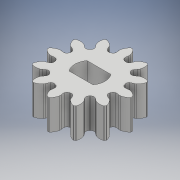
# Autodesk Inventor part: RescueKit-Gear-8
Saved by Autodesk Inventor 2018.3 (Build 223284000, 284)
## iProperties
Created: 2019-03-13
Part Number: RescueKit-Gear-8
Material: 一般
Document SubType Name: Modeling
Designer: shun2
Density: 1 g/cm^3
Appearance: 既定
Author: shun2
Autodesk Inventor part; units mm, degrees
ref_plane "YZ Plane" through (0, 0, 0) normal (1, 0, 0) x (0, 1, 0)
ref_plane "XZ Plane" through (0, 0, 0) normal (0, 1, 0) x (-1, 0, 0)
ref_plane "XY Plane" through (0, 0, 0) normal (0, 0, 1) x (1, 0, 0)
sketch "スケッチ1" plane through (0, 0, 0) normal (0, 0, 1) x (1, 0, 0)
  arc A0 (-0.202, 6.9715) -> (-0.7832, 5.9487) centre (1.1694, 5.5158) ccw
  arc A1 (-0.1354, 6.9987) -> (-0.202, 6.9715) centre (-0.1335, 6.8987) ccw
  arc A2 (0.1354, 6.9987) -> (-0.1354, 6.9987) centre (0, 0) ccw
  arc A3 (0.202, 6.9715) -> (0.1354, 6.9987) centre (0.1335, 6.8987) ccw
  arc A4 (0.7832, 5.9487) -> (0.202, 6.9715) centre (-1.1694, 5.5158) ccw
  arc A5 (0.7831, 5.6009) -> (0.7832, 5.9487) centre (0, 5.775) ccw
  arc A6 (0.7831, 5.6009) -> (0.7441, 5.0639) centre (2.5852, 5.2003) ccw
  arc A7 (0.7441, 5.0639) -> (1.1244, 4.615) centre (1.2427, 5.1008) ccw
  arc A8 (1.3338, 4.5589) -> (1.1244, 4.615) centre (0, 0) ccw
  arc A9 (1.3338, 4.5589) -> (1.8875, 4.7575) centre (1.4742, 5.0388) ccw
  arc A10 (1.8875, 4.7575) -> (2.1223, 5.2421) centre (0.3613, 5.7962) ccw
  arc A11 (2.2961, 5.5433) -> (2.1223, 5.2421) centre (2.8875, 5.0013) ccw
  arc A12 (3.3108, 6.1385) -> (2.2961, 5.5433) centre (3.7707, 4.1921) ccw
  arc A13 (3.3821, 6.1287) -> (3.3108, 6.1385) centre (3.3338, 6.0412) ccw
  arc A14 (3.6166, 5.9933) -> (3.3821, 6.1287) centre (0, 0) ccw
  arc A15 (3.6607, 5.9365) -> (3.6166, 5.9933) centre (3.5649, 5.9077) ccw
  arc A16 (3.6526, 4.7601) -> (3.6607, 5.9365) centre (1.7451, 5.3615) ccw
  arc A17 (3.4786, 4.459) -> (3.6526, 4.7601) centre (2.8875, 5.0013) ccw
  arc A18 (3.4786, 4.459) -> (3.1763, 4.0134) centre (4.839, 3.211) ccw
  arc A19 (3.1763, 4.0134) -> (3.2812, 3.4345) centre (3.6266, 3.7961) ccw
  arc A20 (3.4345, 3.2812) -> (3.2812, 3.4345) centre (0, 0) ccw
  arc A21 (3.4345, 3.2812) -> (4.0134, 3.1763) centre (3.7961, 3.6266) ccw
  arc A22 (4.0134, 3.1763) -> (4.459, 3.4786) centre (3.211, 4.839) ccw
  arc A23 (4.7601, 3.6526) -> (4.459, 3.4786) centre (5.0013, 2.8875) ccw
  arc A24 (5.9365, 3.6607) -> (4.7601, 3.6526) centre (5.3615, 1.7451) ccw
  arc A25 (5.9933, 3.6166) -> (5.9365, 3.6607) centre (5.9077, 3.5649) ccw
  arc A26 (6.1287, 3.3821) -> (5.9933, 3.6166) centre (0, 0) ccw
  arc A27 (6.1385, 3.3108) -> (6.1287, 3.3821) centre (6.0412, 3.3338) ccw
  arc A28 (5.5433, 2.2961) -> (6.1385, 3.3108) centre (4.1921, 3.7707) ccw
  arc A29 (5.2421, 2.1223) -> (5.5433, 2.2961) centre (5.0013, 2.8875) ccw
  arc A30 (5.2421, 2.1223) -> (4.7575, 1.8875) centre (5.7962, 0.3613) ccw
  arc A31 (4.7575, 1.8875) -> (4.5589, 1.3338) centre (5.0388, 1.4742) ccw
  arc A32 (4.615, 1.1244) -> (4.5589, 1.3338) centre (0, 0) ccw
  arc A33 (4.615, 1.1244) -> (5.0639, 0.7441) centre (5.1008, 1.2427) ccw
  arc A34 (5.0639, 0.7441) -> (5.6009, 0.7831) centre (5.2003, 2.5852) ccw
  arc A35 (5.9487, 0.7832) -> (5.6009, 0.7831) centre (5.775, 0) ccw
  arc A36 (6.9715, 0.202) -> (5.9487, 0.7832) centre (5.5158, -1.1694) ccw
  arc A37 (6.9987, 0.1354) -> (6.9715, 0.202) centre (6.8987, 0.1335) ccw
  arc A38 (6.9987, -0.1354) -> (6.9987, 0.1354) centre (0, 0) ccw
  arc A39 (6.9715, -0.202) -> (6.9987, -0.1354) centre (6.8987, -0.1335) ccw
  arc A40 (5.9487, -0.7832) -> (6.9715, -0.202) centre (5.5158, 1.1694) ccw
  arc A41 (5.6009, -0.7831) -> (5.9487, -0.7832) centre (5.775, 0) ccw
  arc A42 (5.6009, -0.7831) -> (5.0639, -0.7441) centre (5.2003, -2.5852) ccw
  arc A43 (5.0639, -0.7441) -> (4.615, -1.1244) centre (5.1008, -1.2427) ccw
  arc A44 (4.5589, -1.3338) -> (4.615, -1.1244) centre (0, 0) ccw
  arc A45 (4.5589, -1.3338) -> (4.7575, -1.8875) centre (5.0388, -1.4742) ccw
  arc A46 (4.7575, -1.8875) -> (5.2421, -2.1223) centre (5.7962, -0.3613) ccw
  arc A47 (5.5433, -2.2961) -> (5.2421, -2.1223) centre (5.0013, -2.8875) ccw
  arc A48 (6.1385, -3.3108) -> (5.5433, -2.2961) centre (4.1921, -3.7707) ccw
  arc A49 (6.1287, -3.3821) -> (6.1385, -3.3108) centre (6.0412, -3.3338) ccw
  arc A50 (5.9933, -3.6166) -> (6.1287, -3.3821) centre (0, 0) ccw
  arc A51 (5.9365, -3.6607) -> (5.9933, -3.6166) centre (5.9077, -3.5649) ccw
  arc A52 (4.7601, -3.6526) -> (5.9365, -3.6607) centre (5.3615, -1.7451) ccw
  arc A53 (4.459, -3.4786) -> (4.7601, -3.6526) centre (5.0013, -2.8875) ccw
  arc A54 (4.459, -3.4786) -> (4.0134, -3.1763) centre (3.211, -4.839) ccw
  arc A55 (4.0134, -3.1763) -> (3.4345, -3.2812) centre (3.7961, -3.6266) ccw
  arc A56 (3.2812, -3.4345) -> (3.4345, -3.2812) centre (0, 0) ccw
  arc A57 (3.2812, -3.4345) -> (3.1763, -4.0134) centre (3.6266, -3.7961) ccw
  arc A58 (3.1763, -4.0134) -> (3.4786, -4.459) centre (4.839, -3.211) ccw
  arc A59 (3.6526, -4.7601) -> (3.4786, -4.459) centre (2.8875, -5.0013) ccw
  arc A60 (3.6607, -5.9365) -> (3.6526, -4.7601) centre (1.7451, -5.3615) ccw
  arc A61 (3.6166, -5.9933) -> (3.6607, -5.9365) centre (3.5649, -5.9077) ccw
  arc A62 (3.3821, -6.1287) -> (3.6166, -5.9933) centre (0, 0) ccw
  arc A63 (3.3108, -6.1385) -> (3.3821, -6.1287) centre (3.3338, -6.0412) ccw
  arc A64 (2.2961, -5.5433) -> (3.3108, -6.1385) centre (3.7707, -4.1921) ccw
  arc A65 (2.1223, -5.2421) -> (2.2961, -5.5433) centre (2.8875, -5.0013) ccw
  arc A66 (2.1223, -5.2421) -> (1.8875, -4.7575) centre (0.3613, -5.7962) ccw
  arc A67 (1.8875, -4.7575) -> (1.3338, -4.5589) centre (1.4742, -5.0388) ccw
  arc A68 (1.1244, -4.615) -> (1.3338, -4.5589) centre (0, 0) ccw
  arc A69 (1.1244, -4.615) -> (0.7441, -5.0639) centre (1.2427, -5.1008) ccw
  arc A70 (0.7441, -5.0639) -> (0.7831, -5.6009) centre (2.5852, -5.2003) ccw
  arc A71 (0.7832, -5.9487) -> (0.7831, -5.6009) centre (0, -5.775) ccw
  arc A72 (0.202, -6.9715) -> (0.7832, -5.9487) centre (-1.1694, -5.5158) ccw
  arc A73 (0.1354, -6.9987) -> (0.202, -6.9715) centre (0.1335, -6.8987) ccw
  arc A74 (-0.1354, -6.9987) -> (0.1354, -6.9987) centre (0, 0) ccw
  arc A75 (-0.202, -6.9715) -> (-0.1354, -6.9987) centre (-0.1335, -6.8987) ccw
  arc A76 (-0.7832, -5.9487) -> (-0.202, -6.9715) centre (1.1694, -5.5158) ccw
  arc A77 (-0.7831, -5.6009) -> (-0.7832, -5.9487) centre (0, -5.775) ccw
  arc A78 (-0.7831, -5.6009) -> (-0.7441, -5.0639) centre (-2.5852, -5.2003) ccw
  arc A79 (-0.7441, -5.0639) -> (-1.1244, -4.615) centre (-1.2427, -5.1008) ccw
  arc A80 (-1.3338, -4.5589) -> (-1.1244, -4.615) centre (0, 0) ccw
  arc A81 (-1.3338, -4.5589) -> (-1.8875, -4.7575) centre (-1.4742, -5.0388) ccw
  arc A82 (-1.8875, -4.7575) -> (-2.1223, -5.2421) centre (-0.3613, -5.7962) ccw
  arc A83 (-2.2961, -5.5433) -> (-2.1223, -5.2421) centre (-2.8875, -5.0013) ccw
  arc A84 (-3.3108, -6.1385) -> (-2.2961, -5.5433) centre (-3.7707, -4.1921) ccw
  arc A85 (-3.3821, -6.1287) -> (-3.3108, -6.1385) centre (-3.3338, -6.0412) ccw
  arc A86 (-3.6166, -5.9933) -> (-3.3821, -6.1287) centre (0, 0) ccw
  arc A87 (-3.6607, -5.9365) -> (-3.6166, -5.9933) centre (-3.5649, -5.9077) ccw
  arc A88 (-3.6526, -4.7601) -> (-3.6607, -5.9365) centre (-1.7451, -5.3615) ccw
  arc A89 (-3.4786, -4.459) -> (-3.6526, -4.7601) centre (-2.8875, -5.0013) ccw
  arc A90 (-3.4786, -4.459) -> (-3.1763, -4.0134) centre (-4.839, -3.211) ccw
  arc A91 (-3.1763, -4.0134) -> (-3.2812, -3.4345) centre (-3.6266, -3.7961) ccw
  arc A92 (-3.4345, -3.2812) -> (-3.2812, -3.4345) centre (0, 0) ccw
  arc A93 (-3.4345, -3.2812) -> (-4.0134, -3.1763) centre (-3.7961, -3.6266) ccw
  arc A94 (-4.0134, -3.1763) -> (-4.459, -3.4786) centre (-3.211, -4.839) ccw
  arc A95 (-4.7601, -3.6526) -> (-4.459, -3.4786) centre (-5.0013, -2.8875) ccw
  arc A96 (-5.9365, -3.6607) -> (-4.7601, -3.6526) centre (-5.3615, -1.7451) ccw
  arc A97 (-5.9933, -3.6166) -> (-5.9365, -3.6607) centre (-5.9077, -3.5649) ccw
  arc A98 (-6.1287, -3.3821) -> (-5.9933, -3.6166) centre (0, 0) ccw
  arc A99 (-6.1385, -3.3108) -> (-6.1287, -3.3821) centre (-6.0412, -3.3338) ccw
  arc A100 (-5.5433, -2.2961) -> (-6.1385, -3.3108) centre (-4.1921, -3.7707) ccw
  arc A101 (-5.2421, -2.1223) -> (-5.5433, -2.2961) centre (-5.0013, -2.8875) ccw
  arc A102 (-5.2421, -2.1223) -> (-4.7575, -1.8875) centre (-5.7962, -0.3613) ccw
  arc A103 (-4.7575, -1.8875) -> (-4.5589, -1.3338) centre (-5.0388, -1.4742) ccw
  arc A104 (-4.615, -1.1244) -> (-4.5589, -1.3338) centre (0, 0) ccw
  arc A105 (-4.615, -1.1244) -> (-5.0639, -0.7441) centre (-5.1008, -1.2427) ccw
  arc A106 (-5.0639, -0.7441) -> (-5.6009, -0.7831) centre (-5.2003, -2.5852) ccw
  arc A107 (-5.9487, -0.7832) -> (-5.6009, -0.7831) centre (-5.775, 0) ccw
  arc A108 (-6.9715, -0.202) -> (-5.9487, -0.7832) centre (-5.5158, 1.1694) ccw
  arc A109 (-6.9987, -0.1354) -> (-6.9715, -0.202) centre (-6.8987, -0.1335) ccw
  arc A110 (-6.9987, 0.1354) -> (-6.9987, -0.1354) centre (0, 0) ccw
  arc A111 (-6.9715, 0.202) -> (-6.9987, 0.1354) centre (-6.8987, 0.1335) ccw
  arc A112 (-5.9487, 0.7832) -> (-6.9715, 0.202) centre (-5.5158, -1.1694) ccw
  arc A113 (-5.6009, 0.7831) -> (-5.9487, 0.7832) centre (-5.775, 0) ccw
  arc A114 (-5.6009, 0.7831) -> (-5.0639, 0.7441) centre (-5.2003, 2.5852) ccw
  arc A115 (-5.0639, 0.7441) -> (-4.615, 1.1244) centre (-5.1008, 1.2427) ccw
  arc A116 (-4.5589, 1.3338) -> (-4.615, 1.1244) centre (0, 0) ccw
  arc A117 (-4.5589, 1.3338) -> (-4.7575, 1.8875) centre (-5.0388, 1.4742) ccw
  arc A118 (-4.7575, 1.8875) -> (-5.2421, 2.1223) centre (-5.7962, 0.3613) ccw
  arc A119 (-5.5433, 2.2961) -> (-5.2421, 2.1223) centre (-5.0013, 2.8875) ccw
  arc A120 (-6.1385, 3.3108) -> (-5.5433, 2.2961) centre (-4.1921, 3.7707) ccw
  arc A121 (-6.1287, 3.3821) -> (-6.1385, 3.3108) centre (-6.0412, 3.3338) ccw
  arc A122 (-5.9933, 3.6166) -> (-6.1287, 3.3821) centre (0, 0) ccw
  arc A123 (-5.9365, 3.6607) -> (-5.9933, 3.6166) centre (-5.9077, 3.5649) ccw
  arc A124 (-4.7601, 3.6526) -> (-5.9365, 3.6607) centre (-5.3615, 1.7451) ccw
  arc A125 (-4.459, 3.4786) -> (-4.7601, 3.6526) centre (-5.0013, 2.8875) ccw
  arc A126 (-4.459, 3.4786) -> (-4.0134, 3.1763) centre (-3.211, 4.839) ccw
  arc A127 (-4.0134, 3.1763) -> (-3.4345, 3.2812) centre (-3.7961, 3.6266) ccw
  arc A128 (-3.2812, 3.4345) -> (-3.4345, 3.2812) centre (0, 0) ccw
  arc A129 (-3.2812, 3.4345) -> (-3.1763, 4.0134) centre (-3.6266, 3.7961) ccw
  arc A130 (-3.1763, 4.0134) -> (-3.4786, 4.459) centre (-4.839, 3.211) ccw
  arc A131 (-3.6526, 4.7601) -> (-3.4786, 4.459) centre (-2.8875, 5.0013) ccw
  arc A132 (-3.6607, 5.9365) -> (-3.6526, 4.7601) centre (-1.7451, 5.3615) ccw
  arc A133 (-3.6166, 5.9933) -> (-3.6607, 5.9365) centre (-3.5649, 5.9077) ccw
  arc A134 (-3.3821, 6.1287) -> (-3.6166, 5.9933) centre (0, 0) ccw
  arc A135 (-3.3108, 6.1385) -> (-3.3821, 6.1287) centre (-3.3338, 6.0412) ccw
  arc A136 (-2.2961, 5.5433) -> (-3.3108, 6.1385) centre (-3.7707, 4.1921) ccw
  arc A137 (-2.1223, 5.2421) -> (-2.2961, 5.5433) centre (-2.8875, 5.0013) ccw
  arc A138 (-2.1223, 5.2421) -> (-1.8875, 4.7575) centre (-0.3613, 5.7962) ccw
  arc A139 (-1.8875, 4.7575) -> (-1.3338, 4.5589) centre (-1.4742, 5.0388) ccw
  arc A140 (-1.1244, 4.615) -> (-1.3338, 4.5589) centre (0, 0) ccw
  arc A141 (-1.1244, 4.615) -> (-0.7441, 5.0639) centre (-1.2427, 5.1008) ccw
  arc A142 (-0.7441, 5.0639) -> (-0.7831, 5.6009) centre (-2.5852, 5.2003) ccw
  arc A143 (-0.7832, 5.9487) -> (-0.7831, 5.6009) centre (0, 5.775) ccw
  line L0 (-2, 1.5) -> (2, 1.5)
  line L1 (2, -1.5) -> (-2, -1.5)
  arc A144 (-2, 1.5) -> (-2, -1.5) centre (0, 0) ccw
  arc A145 (2, -1.5) -> (2, 1.5) centre (0, 0) ccw
  point P0 (0, 0)
  point P1 (0, 0)
  constraints: 292 point on circle, 146 centre point, 4 end point, 1 coincident, 1 horizontal, 1 parallel
extrude "押し出し1" add sketch "スケッチ1" along normal blind 5
